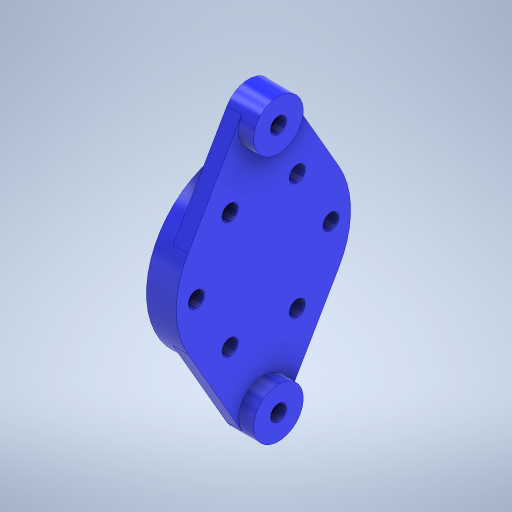
# Autodesk Inventor part: endeff_3dp2
Saved by Autodesk Inventor 2024 (Build 280153000, 153)
## iProperties
Created: 2024-12-13
Part Number: endeff_3dp2
Material: ABS プラスチック
Document SubType Name: Modeling
Designer: hirek
Density: 1.06 g/cm^3
Appearance: 青 - 壁塗料 - 光沢
Author: hirek
Autodesk Inventor part; units mm, degrees
ref_plane "YZ Plane" through (0, 0, 0) normal (1, 0, 0) x (0, 1, 0)
ref_plane "XZ Plane" through (0, 0, 0) normal (0, 1, 0) x (-1, 0, 0)
ref_plane "XY Plane" through (0, 0, 0) normal (0, 0, 1) x (1, 0, 0)
sketch "スケッチ1" plane through (0, 0, 0) normal (1, 0, 0) x (0, 1, 0)
  circle A0 centre (0, 0) radius 17.5
  dimension "d0" = 35
  constraints: 1 centre point, 1 coincident
  measures "d0" diameter of A0
extrude "押し出し1" add sketch "スケッチ1" along normal blind 3
sketch "スケッチ2" plane through (3, 0, 0) normal (1, 0, 0) x (0, 0, -1)
  circle A0 centre (0, 0) radius 13.5
  point P0 (13.5, 0)
  point P1 (6.75, 11.6913)
  point P2 (-6.75, 11.6913)
  point P3 (-13.5, 0)
  point P4 (-6.75, -11.6913)
  point P5 (6.75, -11.6913)
  dimension "d3" = 27
  dimension "d6" = 360
  constraints: 1 coincident, 1 horizontal alignment, 9 other
hole "穴1" at (3, 0, -13.5) at (3, 11.6913, -6.75) at (3, 11.6913, 6.75) at (3, 0, 13.5) at (3, -11.6913, 6.75) at (3, -11.6913, -6.75) direction (-1, 0, 0) diameter 3.2 end through all
sketch "スケッチ4" plane through (3, 0, 0) normal (1, 0, 0) x (0, 0, -1)
  circle A0 centre (0, 0) radius 25
  circle A1 centre (0, -25) radius 5
  circle A2 centre (0, 25) radius 5
  circle A3 centre (13.5, 0) radius 1.6 projected
  circle A4 centre (-13.5, 0) radius 1.6 projected
  line L0 (-1.8583, 31.7813) -> (-19.7652, 0.7657)
  line L1 (-19.9094, -0.516) -> (-0.3337, -34.4219)
  line L2 (1.1974, -32.9261) -> (19.8479, -0.6225)
  line L3 (2.1736, 31.2353) -> (21.8646, -2.8706)
  circle A5 centre (0, 0) radius 17.5 projected
  point P0 (-4.3301, 27.5)
  point P1 (-15.1554, 8.75)
  point P2 (-15.1554, -8.75)
  point P3 (-4.3301, -27.5)
  point P4 (4.3301, -27.5)
  point P5 (15.1554, -8.75)
  point P6 (15.1554, 8.75)
  point P7 (4.3301, 27.5)
  dimension "d22" = 50
  dimension "d23" = 10
  dimension "d24" = 10
  dimension "d25" = 13.5
  dimension "d26" = 13.5
  constraints: 8 end point, 8 tangent, 3 centre point, 2 point on circle, 1 coincident
  measures "d22" diameter of A0
  measures "d23" diameter of A1
  measures "d24" diameter of A2
  measures "d25" horizontal distance of A3.centre A2.centre
  measures "d26" horizontal distance of A4.centre A1.centre
extrude "押し出し2" add sketch "スケッチ4" along normal blind 3 contours L3 A5 L0 A0 A2 | A0 A2 L3 | L2 A1 A0 | A0 A1 L1 A5 L2 | A2 A0 | A0 A2 | A5 | A1 A0 | A0 A1 | A0 L0 A2 | A1 L1 A0 | A3 | A4
sketch "スケッチ6" plane through (6, 0, 0) normal (1, 0, 0) x (0, 0, -1)
  arc A0 (4.3301, 27.5) -> (-4.3301, 27.5) centre (0, 25) ccw projected
  circle A1 centre (0, 25) radius 5
  arc A2 (-4.3301, -27.5) -> (4.3301, -27.5) centre (0, -25) ccw projected
  circle A3 centre (0, -25) radius 5
  point P0 (0, 0)
  point P1 (-4.3301, 27.5)
  point P2 (4.3301, 27.5)
  dimension "d29" = 10
  dimension "d30" = 10
  constraints: 2 centre point, 2 coincident
  measures "d29" diameter of A1
  measures "d30" diameter of A3
extrude "押し出し3" add sketch "スケッチ6" along normal blind 3
sketch "スケッチ7" plane through (0, 0, 0) normal (-1, 0, 0) x (0, 0, 1)
  circle A0 centre (6.75, 11.6913) radius 1.6 projected
  circle A1 centre (13.5, 0) radius 1.6 projected
  circle A2 centre (6.75, -11.6913) radius 1.6 projected
  circle A3 centre (-6.75, -11.6913) radius 1.6 projected
  circle A4 centre (-13.5, 0) radius 1.6 projected
  circle A5 centre (-6.75, 11.6913) radius 1.6 projected
  arc A6 (4.3301, 27.5) -> (-4.3301, 27.5) centre (0, 25) ccw projected
  arc A7 (-4.3301, -27.5) -> (4.3301, -27.5) centre (0, -25) ccw projected
  point P0 (0, 0)
  constraints: 8 coincident
hole "穴2" at (0, 11.6913, 6.75) at (0, 0, 13.5) at (0, -11.6913, 6.75) at (0, -11.6913, -6.75) at (0, 0, -13.5) at (0, 11.6913, -6.75) at (0, 25, 0) at (0, -25, 0) direction (1, 0, 0) diameter 3.2 end through all
sketch "スケッチ9" plane through (0, 0, 0) normal (-1, 0, 0) x (0, 0, 1)
  circle A0 centre (0, 25) radius 1.6 projected
  circle A1 centre (0, 25) radius 3.5
  circle A2 centre (0, -25) radius 1.6 projected
  circle A3 centre (0, -25) radius 3.5
  point P0 (0, 0)
  point P1 (0.5822, 17.4903)
  point P2 (-0.5822, 17.4903)
  point P3 (-0.5822, -17.4903)
  point P4 (0.5822, -17.4903)
  dimension "d40" = 7
  dimension "d41" = 7
  constraints: 2 centre point, 2 coincident, 2 other
  measures "d40" diameter of A1
  measures "d41" diameter of A3
extrude "押し出し4" cut sketch "スケッチ9" against normal blind 7 contours A0 | A1 | A2 | A3
